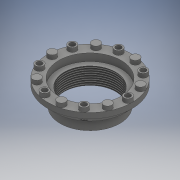
# Autodesk Inventor part: entraineur sur roue libre
Saved by Autodesk Inventor 2018.1 (Build 221171000, 171)
## iProperties
Created: 2022-06-03
Part Number: entraineur sur roue libre
Material: Generic
Document SubType Name: Modeling
Designer: mouta
Density: 1 g/cm^3
Appearance: Default
Author: mouta
Autodesk Inventor part; units mm, degrees
ref_plane "YZ Plane" through (0, 0, 0) normal (1, 0, 0) x (0, 1, 0)
ref_plane "XZ Plane" through (0, 0, 0) normal (0, 1, 0) x (-1, 0, 0)
ref_plane "XY Plane" through (0, 0, 0) normal (0, 0, 1) x (1, 0, 0)
sketch "Sketch1" plane through (0, 0, 0) normal (0, 1, 0) x (-1, 0, 0)
  line L0 (0, 0) -> (0, -23.6629)
  line L1 (0, 0) -> (19, 0)
  line L2 (19, -5.5) -> (19, -18)
  line L3 (19, -18) -> (22, -18)
  line L4 (22, -18) -> (22, -9)
  line L5 (22, -9) -> (26, -9)
  line L6 (31, -4) -> (31, 0)
  line L7 (31, 0) -> (23, 0)
  line L8 (23, 0) -> (23, -5.5)
  line L9 (23, -5.5) -> (19, -5.5)
  line L10 (26, -9) -> (26, -9)
  line L11 (26, -9) -> (31, -9)
  line L12 (31, 0) -> (31, -4)
  line L13 (31, -4) -> (26, -9)
  dimension "d0" = 19
  dimension "d1" = 18
  dimension "d2" = 3
  dimension "d5" = 8
  dimension "d13" = 5.5
  dimension "d15" = 9
  dimension "d24" = 12.5
  dimension "d92" = 0
  dimension "d93" = 4
  dimension "d95" = 135
  constraints: 28 end point, 9 perpendicular, 2 point on line, 1 horizontal, 1 vertical
  measures "d0" distance of L0.start L1.end
  measures "d1" distance of L1.end L2.end
  measures "d2" distance of L2.end L3.end
  measures "d5" distance of L6.end L7.end
  measures "d13" distance of L7.end L8.end
  measures "d15" distance of L11.end L6.end
  measures "d24" distance of L2.start L2.end
  measures "d92" distance of L10.end L5.end
  measures "d93" distance of L6.start L6.end
  measures "d95" angle of L12 L13
revolve "Revolution1" add sketch "Sketch1" angle 360 about axis through (0, 0, 0) along (0, 0, -1)
thread "Thread1" size "M38x1.5" class "6H" standard "ANSI Metric M Profile" full length
sketch "Sketch2" plane through (0, 0, 0) normal (0, 0, 1) x (1, 0, 0)
  line L0 (0, 0) -> (28, 0)
  circle A0 centre (28, 0) radius 3
  circle A1 centre (25.2271, -12.1487) radius 3
  circle A2 centre (17.4577, -21.8913) radius 3
  circle A3 centre (6.2306, -27.298) radius 3
  circle A4 centre (-6.2306, -27.298) radius 3
  circle A5 centre (-17.4577, -21.8913) radius 3
  circle A6 centre (-25.2271, -12.1487) radius 3
  circle A7 centre (-28, 0) radius 3
  circle A8 centre (-25.2271, 12.1487) radius 3
  circle A9 centre (-17.4577, 21.8913) radius 3
  circle A10 centre (-6.2306, 27.298) radius 3
  circle A11 centre (6.2306, 27.298) radius 3
  circle A12 centre (17.4577, 21.8913) radius 3
  circle A13 centre (25.2271, 12.1487) radius 3
  dimension "d16" = 28
  dimension "d17" = 6
  dimension "d20" = 360
  constraints: 14 centre point, 3 coincident, 2 end point, 1 horizontal, 40 other
  measures "d16" distance of L0.start L0.end
  measures "d17" diameter of A0
extrude "Extrusion2" add sketch "Sketch2" along normal blind 3
hole "Hole1" at (-25.2271, 12.1487, 3) direction (0, 0, -1) diameter 4 depth 10 tip angle 118
hole "Hole2" at (-6.2306, 27.298, 3) direction (0, 0, -1) diameter 4 depth 10 tip angle 118
hole "Hole3" at (-25.2271, -12.1487, 3) direction (0, 0, -1) diameter 4 depth 10 tip angle 118
hole "Hole4" at (-6.2306, -27.298, 3) direction (0, 0, -1) diameter 4 depth 10 tip angle 118
hole "Hole5" at (17.4577, -21.8913, 3) direction (0, 0, -1) diameter 4 depth 10 tip angle 118
hole "Hole6" at (28, 0, 3) direction (0, 0, -1) diameter 4 depth 10 tip angle 118
hole "Hole7" at (17.4577, 21.8913, 3) direction (0, 0, -1) diameter 4 depth 10 tip angle 118
body "Solid1"
